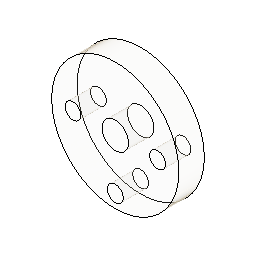
AssemblyStatorSpacer v5 (Autodesk Fusion 360 archive; units mm, degrees)
design "StatorSpacer"
Autodesk Fusion 360 part; units mm, degrees
sketch "Sketch1" plane through (0, 0, 0) normal (0, 1, 0) x (1, 0, 0)
  circle A0 centre (0, 0) radius 12
  circle A1 centre (0, 0) radius 9.5 construction
  circle A2 centre (0, 0) radius 8 construction
  line L0 (0, 0) -> (0, -9.5) construction
  line L1 (0, 0) -> (0, 9.5) construction
  line L2 (0, 0) -> (8, 0) construction
  line L3 (0, 0) -> (-8, 0) construction
  circle A3 centre (0, 9.5) radius 1.5
  circle A4 centre (8, 0) radius 1.5
  circle A5 centre (-8, 0) radius 1.5
  circle A6 centre (0, 0) radius 2.5
  dimension "d1" = 24
  dimension "d2" = 19
  dimension "d3" = 16
  dimension "d5" = 3
  dimension "d6" = 3
  dimension "d7" = 3
  dimension "d10" = 5
  constraint coincident A0.centre A1.centre
  constraint concentric A0 A1
  constraint coincident A1 L0.end
  constraint vertical L0
  constraint coincident A1 L1.end
  constraint parallel L0 L1
  constraint coincident A2 L2.end
  constraint perpendicular L0 L2
  constraint coincident A2 L3.end
  constraint perpendicular L0 L3
  constraint coincident L1.end A3.centre
  constraint coincident L2.end A4.centre
  constraint coincident L3.end A5.centre
  constraint concentric A0 A6
  measures "d1" diameter of A0
  measures "d2" diameter of A1
  measures "d3" diameter of A2
  measures "d5" diameter of A3
  measures "d6" diameter of A4
  measures "d7" diameter of A5
  measures "d10" diameter of A6
extrude "Extrude1" add sketch "Sketch1" along normal blind 4.8
